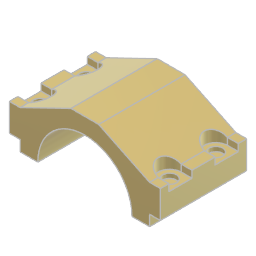
Weird lookingbridge thingy (Autodesk Fusion 360 design; units mm, degrees)
Autodesk Fusion 360 part; units mm, degrees
sketch "Sketch1" plane through (0, 0, 0) normal (0, 0, 1) x (1, 0, 0)
  line L0 (-30.5, 0) -> (-42, 0)
  line L1 (30.5, 0) -> (42, 0)
  line L2 (-42, 0) -> (-42, 7)
  line L3 (-42, 7) -> (-49, 7)
  line L4 (-49, 7) -> (-49, 25)
  line L5 (-49, 25) -> (-42, 25)
  line L6 (42, 0) -> (42, 7)
  line L7 (42, 7) -> (49, 7)
  line L8 (49, 7) -> (49, 25)
  line L9 (49, 25) -> (42, 25)
  line L10 (0, 0) -> (0, 41) construction
  line L11 (0, 41) -> (9, 41)
  line L12 (0, 41) -> (-9, 41)
  line L13 (9, 41) -> (42, 25)
  line L14 (-9, 41) -> (-42, 25)
  arc A0 (30.5, 0) -> (-30.5, 0) centre (0, 0) ccw
  dimension "d1" = 42
  dimension "d2" = 42
  dimension "d3" = 7
  dimension "d4" = 7
  dimension "d5" = 18
  dimension "d6" = 7
  dimension "d7" = 7
  dimension "d8" = 18
  dimension "d9" = 7
  dimension "d10" = 41
  dimension "d11" = 9
  dimension "d12" = 9
  dimension "d13" = 61
  constraint horizontal L0
  constraint parallel L0 L1
  constraint perpendicular L0 L2
  constraint perpendicular L2 L3
  constraint perpendicular L3 L4
  constraint perpendicular L4 L5
  constraint perpendicular L1 L6
  constraint perpendicular L6 L7
  constraint perpendicular L7 L8
  constraint perpendicular L8 L9
  constraint coincident L10.start A0.centre
  constraint perpendicular L1 L10
  constraint perpendicular L10 L11
  constraint perpendicular L10 L12
  measures "d1" distance of L10.start L0.end
  measures "d2" distance of L10.start L1.end
  measures "d3" distance of L0.end L2.end
  measures "d4" distance of L2.end L3.end
  measures "d5" distance of L3.end L4.end
  measures "d6" distance of L1.end L6.end
  measures "d7" distance of L6.end L7.end
  measures "d8" distance of L7.end L8.end
  measures "d9" distance of L8.end L9.end
  measures "d10" distance of L10.start L10.end
  measures "d11" distance of L10.end L11.end
  measures "d12" distance of L10.end L12.end
  measures "d13" diameter of A0
extrude "Extrude1" add sketch "Sketch1" against normal blind 56
sketch "Sketch2" plane through (0, 0, 0) normal (0, 1, 0) x (1, 0, 0)
ref_plane "WorkPlane1" through (0, 20.5, 0) normal (0, 1, 0) x (0, 0, 1)
sketch "Sketch3" plane through (0, 20.5, 0) normal (0, 1, 0) x (1, 0, 0)
  line L0 (0, 0) -> (-49, 0)
  line L1 (-49, 0) -> (49, 0)
  line L2 (49, 0) -> (49, 56)
  line L3 (49, 56) -> (-49, 56)
  line L4 (-49, 56) -> (-49, 0)
  line L5 (0, 0) -> (-9, 0)
  line L6 (0, 0) -> (9, 0)
  line L7 (-9, 0) -> (-9, 56)
  line L8 (9, 0) -> (9, 56)
  line L9 (-49, 0) -> (-49, 28) construction
  line L10 (-49, 28) -> (49, 28) construction
  line L11 (49, 28) -> (49, 43) construction
  line L12 (49, 43) -> (-49, 43) construction
  line L13 (-49, 28) -> (-49, 13) construction
  line L14 (-49, 13) -> (49, 13) construction
  line L15 (49, 0) -> (41.09, 0)
  line L16 (41.09, 0) -> (41.09, 56) construction
  line L17 (-49, 0) -> (-41.09, 0) construction
  line L18 (-41.09, 0) -> (-41.09, 56) construction
  line L19 (-41.09, 0) -> (-42, 0) construction
  line L20 (-42, 0) -> (-42, 56) construction
  line L21 (49, 0) -> (42, 0) construction
  line L22 (42, 0) -> (42, 56) construction
  circle A0 centre (42, 43) radius 4.5
  circle A1 centre (42, 13) radius 4.5
  circle A2 centre (-42, 13) radius 4.5
  circle A3 centre (-42, 43) radius 4.5
  line L23 (-42, 20.5) -> (-49, 20.5)
  line L24 (-42, 5.5) -> (-49, 5.5466)
  arc A4 (-42.0998, 5.5007) -> (-42, 20.5) centre (-42, 13) ccw
  arc A5 (-42, 35.5) -> (-42, 50.5) centre (-42, 43) ccw
  line L25 (-42, 50.5) -> (-49, 50.5)
  line L26 (-42, 35.5) -> (-49, 35.5)
  line L27 (42, 50.5) -> (49, 50.5)
  line L28 (42, 35.5) -> (49, 35.5)
  line L29 (42, 20.5) -> (49, 20.5)
  line L30 (42, 5.5) -> (49, 5.5)
  arc A6 (42, 20.5) -> (42, 5.5) centre (42, 13) ccw
  arc A7 (42, 50.5) -> (42, 35.5) centre (42, 43) ccw
  dimension "d17" = 49
  dimension "d18" = 98
  dimension "d19" = 56
  dimension "d20" = 9
  dimension "d21" = 9
  dimension "d22" = 15
  dimension "d23" = 7.91
  dimension "d24" = 7.91
  dimension "d25" = 7
  dimension "d26" = 9
  dimension "d27" = 15
  dimension "d28" = 9
  dimension "d29" = 15
  dimension "d30" = 9
  dimension "d31" = 15
  dimension "d32" = 9
  dimension "d33" = 15
  constraint coincident L0.start L5.start
  constraint horizontal L0
  constraint horizontal L1
  constraint vertical L2
  constraint horizontal L3
  constraint vertical L4
  constraint parallel L0 L5
  constraint parallel L1 L6
  constraint coincident L3 L7.end
  constraint perpendicular L3 L7
  constraint coincident L3 L8.end
  constraint perpendicular L3 L8
  constraint midpoint L4 L9.end
  constraint midpoint L2 L10.end
  constraint coincident L2 L11.end
  constraint coincident L4 L12.end
  constraint perpendicular L4 L12
  constraint coincident L4 L13.end
  constraint perpendicular L10 L13
  constraint coincident L2 L14.end
  constraint perpendicular L2 L14
  constraint perpendicular L2 L15
  constraint coincident L3 L16.end
  constraint perpendicular L3 L16
  constraint perpendicular L4 L17
  constraint coincident L3 L18.end
  constraint perpendicular L3 L18
  constraint coincident L0 L19.end
  constraint coincident L3 L20.end
  constraint perpendicular L3 L20
  constraint perpendicular L2 L21
  constraint coincident L3 L22.end
  constraint perpendicular L3 L22
  constraint coincident L12 A0.centre
  constraint coincident L22 A0.centre
  constraint concentric A0 A7
  constraint coincident L14 A1.centre
  constraint coincident L22 A1.centre
  constraint concentric A1 A6
  constraint coincident L20 A2.centre
  constraint coincident L14 A2.centre
  constraint concentric A2 A4
  constraint coincident L20 A3.centre
  constraint coincident L12 A3.centre
  constraint concentric A3 A5
  constraint coincident L20 L23.start
  constraint midpoint L13 L23.end
  constraint coincident L24.start A4
  constraint coincident L20 L24.start
  constraint coincident L9 L24.end
  constraint coincident L24 A4.start
  constraint coincident L20 A5.end
  constraint coincident L4 L25.end
  constraint tangent A5 L25
  constraint coincident L20 A5.start
  constraint tangent A5 L26
  constraint coincident L22 L27.start
  constraint coincident L2 L27.end
  constraint tangent L27 A7
  constraint coincident L22 L28.start
  constraint midpoint L11 L28.end
  constraint coincident L22 L29.start
  constraint coincident L2 L29.end
  constraint tangent L29 A6
  constraint coincident L22 L30.start
  constraint coincident L2 L30.end
  constraint tangent L30 A6
  measures "d17" distance of L0.start L0.end
  measures "d18" distance of L0.end L1.end
  measures "d19" distance of L0.end L3.end
  measures "d20" distance of L0.start L5.end
  measures "d21" distance of L0.start L6.end
  measures "d22" distance of L10.end L11.end
  measures "d23" distance of L1.end L15.end
  measures "d24" distance of L0.end L17.end
  measures "d25" distance of L1.end L21.end
  measures "d26" diameter of A0
  measures "d27" diameter of A7
  measures "d28" diameter of A1
  measures "d29" diameter of A6
  measures "d30" diameter of A2
  measures "d31" diameter of A4
  measures "d32" diameter of A3
  measures "d33" diameter of A5
extrude "Extrude2" cut sketch "Sketch3" along normal blind 32 contours A0 | A1 | A2 | A3
extrude "Extrude3" cut sketch "Sketch3" along normal blind 14 contours L4 L23 L24 A4 | L4 A5 L25 L26 | L2 L29 L30 A6 | L2 L27 L28 A7
extrude "Extrude4" cut sketch "Sketch3" against normal blind 3 contours A0 | A1 | A2 | A3
move_body "Move1" bodies 1 to x (1, 0, 0) y (0, 1, 0) z (0, 0, 1) at (0, 0, 35)
